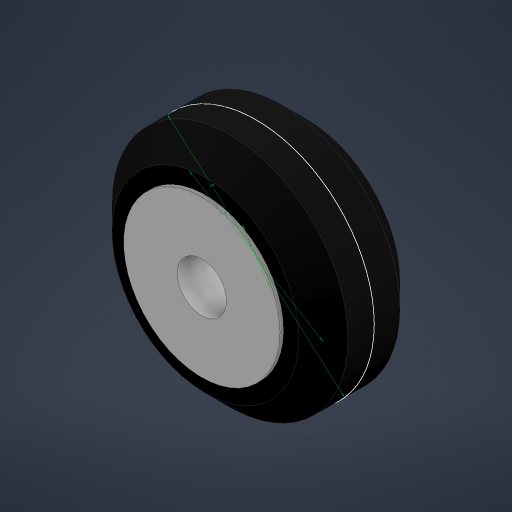
# Autodesk Inventor part: Printer Wheel
Saved by Autodesk Inventor 2024.2 (Build 282272000, 272)
## iProperties
Created: 2024-10-16
Part Number: Printer Wheel
Material: Generic
Document SubType Name: Modeling
Designer: jerem
Density: 1 g/cm^3
Appearance: Default
Author: jerem
Autodesk Inventor part; units mm, degrees
ref_plane "YZ Plane" through (0, 0, 0) normal (1, 0, 0) x (0, 1, 0)
ref_plane "XZ Plane" through (0, 0, 0) normal (0, 1, 0) x (-1, 0, 0)
ref_plane "XY Plane" through (0, 0, 0) normal (0, 0, 1) x (1, 0, 0)
sketch "Sketch1" plane through (0, 0, 0) normal (0, 0, 1) x (1, 0, 0)
  circle A0 centre (0, 0) radius 2.5
  circle A1 centre (0, 0) radius 12
  circle A2 centre (0, 0) radius 7.95
  dimension "d0" = 5
  dimension "d1" = 24
  dimension "d2" = 15.9
  constraints: 3 centre point, 3 coincident
  measures "d0" diameter of A0
  measures "d1" diameter of A1
  measures "d2" diameter of A2
extrude "Extrusion1" add sketch "Sketch1" along normal mid plane 11 contours A2
extrude "Extrusion2" add sketch "Sketch1" along normal mid plane 10.3 contours A1
chamfer "Chamfer1" distance 2.5 angle 45 2 edges at (-12, 0, 5.15) (-12, 0, -5.15)
body "Solid1"
